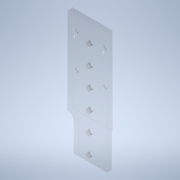
# Autodesk Inventor part: Plate
Saved by Autodesk Inventor 2022 (Build 260153000, 153)
## iProperties
Created: 2022-02-10
Part Number: Plate
Material: PET Plastic
Document SubType Name: Modeling
Designer: br4ch
Density: 1.541 g/cm^3
Appearance: Polycarbonate - Clear
Author: br4ch
Autodesk Inventor part; units mm, degrees
ref_plane "YZ Plane" through (0, 0, 0) normal (1, 0, 0) x (0, 1, 0)
ref_plane "XZ Plane" through (0, 0, 0) normal (0, 1, 0) x (-1, 0, 0)
ref_plane "XY Plane" through (0, 0, 0) normal (0, 0, 1) x (1, 0, 0)
sketch "Sketch1" plane through (0, 0, 0) normal (0, 0, 1) x (1, 0, 0)
  line L0 (-146.5, 49) -> (-146.5, 125.5)
  line L1 (-146.5, 125.5) -> (-111.5, 125.5)
  line L2 (-111.5, 125.5) -> (-111.5, 19)
  line L3 (-111.5, 19) -> (-141, 19)
  line L4 (-141, 19) -> (-141, 43.5)
  arc A0 (-141, 43.5) -> (-146.5, 49) centre (-146.5, 43.5) ccw
  line L5 (-129, 13.9597) -> (-129, 176.9597)
  circle A1 centre (-129, 23) radius 1.9
  circle A2 centre (-129, 40) radius 1.9
  circle A3 centre (-129, 57) radius 1.9
  circle A4 centre (-129, 74) radius 1.9
  circle A5 centre (-129, 91) radius 1.9
  circle A6 centre (-129, 108) radius 1.9
  circle A7 centre (-141.5, 80.5) radius 3.3
  circle A8 centre (-141.5, 80.5) radius 1.6
  line L6 (-154.2414, 80.5) -> (-103.7586, 80.5) construction
  circle A9 centre (-141.5, 110.5) radius 1.6
  circle A10 centre (-141.5, 110.5) radius 3.3
  circle A11 centre (-116.5, 80.5) radius 3.3
  circle A12 centre (-116.5, 80.5) radius 1.6
  circle A13 centre (-116.5, 110.5) radius 1.6
  circle A14 centre (-116.5, 110.5) radius 3.3
  line L7 (-146.5, 49) -> (-111.5, 49)
  point P0 (0, 0)
  dimension "d0" = 5.5
  dimension "d1" = 76.5
  dimension "d2" = 35
  dimension "d3" = 106.5
  dimension "d5" = 17.5
  dimension "d6" = 3.8
  dimension "d9" = 17
  dimension "d14" = 85
  dimension "d15" = 4
  dimension "d16" = 6.6
  dimension "d17" = 3.2
  dimension "d20" = 30
  dimension "d25" = 30
  dimension "d53" = 5
  dimension "d54" = 15
  constraints: 16 end point, 15 centre point, 6 perpendicular, 5 symmetric about line, 4 coincident, 4 vertical, 3 point on line, 2 point on circle, 1 line through centre, 1 tangent, 18 other
  measures "d0" radius of A0
  measures "d1" distance of L0.start L0.end
  measures "d2" distance of L0.end L1.end
  measures "d3" distance of L1.end L2.end
  measures "d5" distance between parallel lines of L5 L2
  measures "d6" diameter of A1
  measures "d9" distance of A1.centre A2.centre
  measures "d14" distance of A6.centre A1.centre
  measures "d15" distance from line of L3 A1.centre
  measures "d16" diameter of A7
  measures "d17" diameter of A8
  measures "d20" distance of A8.centre A9.centre
  measures "d25" distance between parallel lines of L3 L7
  measures "d53" distance from line of L0 A9.centre
  measures "d54" distance from line of L1 A9.centre
extrude "Extrusion1" add sketch "Sketch1" against normal blind 4.5 contours L0 L1 L5 A6 A5 A4 A3 L7 | L5 A3 A4 A5 A6 L1 L2 L7 | A7 | A10 | A11 | A14
sketch "Sketch2" plane through (0, 0, 0) normal (0, 0, 1) x (1, 0, 0)
  circle A0 centre (-141.5, 80.5) radius 1.6 projected
  circle A1 centre (-141.5, 110.5) radius 1.6 projected
  circle A2 centre (-116.5, 110.5) radius 1.6 projected
  circle A3 centre (-116.5, 80.5) radius 1.6 projected
  point P0 (0, 0)
  constraints: 4 coincident
hole "Hole1" at (-141.5, 80.5, 0) at (-141.5, 110.5, 0) at (-116.5, 110.5, 0) at (-116.5, 80.5, 0) direction (0, 0, -1) diameter 3.2 end through all countersink diameter 6.6 countersink angle 90
extrude "Extrusion2" add sketch "Sketch1" against normal blind 4 contours L7 L5 A2 A1 L3 L4 A0 | L7 L2 L3 L5 A1 A2
chamfer "Chamfer1" distance 0.5 angle 45 6 edges at (-130.9, 108, 0) (-130.9, 91, 0) (-130.9, 74, 0) (-130.9, 57, 0) (-130.9, 40, 0) (-130.9, 23, 0) measured on face at (-131.4, 74, 0) measured on face at (-131.4, 91, 0) measured on face at (-131.4, 108, 0) measured on face at (-131.4, 23, 0) measured on face at (-131.4, 40, 0) measured on face at (-131.4, 57, 0)
thread "Thread1" size "M4x0.7" class "6H" standard "ISO Metric profile" full length
thread "Thread2" size "M4x0.7" class "6H" standard "ANSI Metric M Profile" full length
thread "Thread3" size "M4x0.7" class "6H" standard "ANSI Metric M Profile" full length
thread "Thread4" size "M4x0.7" class "6H" standard "ANSI Metric M Profile" full length
thread "Thread5" size "M4x0.7" class "6H" standard "ANSI Metric M Profile" full length
thread "Thread6" size "M4x0.7" class "6H" standard "ANSI Metric M Profile" full length
ref_plane "Work Plane1" through (-129, 13.9597, 0) normal (1, 0, 0) x (0, 1, 0)
equation "\"d6\" = m4"
equation "\"m3\" = 2.8"
equation "\"m4\" = 3.8"
body "Solid1"
